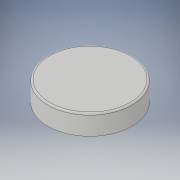
# Autodesk Inventor part: CCF
Saved by Autodesk Inventor 2018 (Build 220112000, 112)
## iProperties
Created: 2017-07-31
Part Number: CCF
Material: Generic
Document SubType Name: Modeling
Designer: Nour Kanso
Density: 1 g/cm^3
Appearance: Default
Author: Nour Kanso
Autodesk Inventor part; units mm, degrees
ref_plane "YZ Plane" through (0, 0, 0) normal (1, 0, 0) x (0, 1, 0)
ref_plane "XZ Plane" through (0, 0, 0) normal (0, 1, 0) x (-1, 0, 0)
ref_plane "XY Plane" through (0, 0, 0) normal (0, 0, 1) x (1, 0, 0)
sketch "Sketch5" plane through (0, 0, 0) normal (0, 1, 0) x (-1, 0, 0)
  circle A0 centre (0, 0) radius 32.131
  dimension "d28" = 64.262
  constraints: 1 centre point, 1 coincident
  measures "d28" diameter of A0
extrude "Extrusion3" add sketch "Sketch5" along normal blind 15.24
fillet "Fillet2" radius 1.27 1 edges at (32.131, 15.24, 0)
shell "Shell5" thickness 1.27 removed faces 1 at (-12.2357, 0, 10.0143)
thread "Thread6" size "2 1/2-4 UNC" class "2B" standard "ANSI Unified Screw Threads" full length
sketch "Sketch14" plane through (0, 13.97, 30.861) normal (-1, 0, 0) x (0, -1, 0)
  line L0 (-3.762, -0.339) -> (-3.1751, -0.339) construction
  line L1 (0.5868, -3.8052) -> (-0.0001, -4.8217) construction
  line L2 (-6.3501, -4.8217) -> (-6.937, -3.8052) construction
  line L3 (-2.5882, -0.339) -> (-3.1751, 0.6775) construction
  line L4 (-3.1751, 0.6775) -> (-3.762, -0.339) construction
  line L5 (-6.3501, -4.8217) -> (-5.7632, -3.8052) construction
  line L6 (-2.5882, -0.339) -> (-0.587, -3.8052)
  line L7 (-6.937, -3.8052) -> (-5.7632, -3.8052) construction
  arc A0 (-6.937, -3.8052) -> (-6.3501, -4.1441) centre (-6.3501, -3.4664) ccw construction
  line L8 (0.5868, -3.8052) -> (-0.587, -3.8052) construction
  line L9 (-6.3501, -4.8217) -> (-6.3501, -3.8052) construction
  line L10 (-0.0001, -4.8217) -> (-0.0001, -3.8052) construction
  line L11 (-3.1751, 0.6775) -> (-3.1751, -0.0002) construction
  line L12 (-6.3501, -4.1441) -> (-0.0001, -4.1441)
  arc A1 (-6.3501, -4.1441) -> (-5.7632, -3.8052) centre (-6.3501, -3.4664) ccw
  line L13 (-0.587, -3.8052) -> (-0.0001, -4.8217) construction
  line L14 (-5.7632, -3.8052) -> (-3.762, -0.339)
  line L15 (-0.0001, -0.0002) -> (-0.0001, 0.0177)
  line L16 (-0.0001, 0.0177) -> (-0.0001, -0.0002)
  line L17 (-0.0001, -0.0002) -> (0.0334, -0.0002)
  arc A2 (-0.587, -3.8052) -> (-0.0001, -4.1441) centre (-0.0001, -3.4664) ccw
  arc A3 (-0.0001, -4.1441) -> (0.5868, -3.8052) centre (-0.0001, -3.4664) ccw construction
  arc A4 (-3.1751, -0.0002) -> (-3.762, -0.339) centre (-3.1751, -0.6779) ccw
  arc A5 (-2.5882, -0.339) -> (-3.1751, -0.0002) centre (-3.1751, -0.6779) ccw
  line L18 (-3.1751, -0.0002) -> (-3.1751, -0.339) construction
  line L19 (-3.1751, -0.339) -> (-2.5882, -0.339) construction
  dimension "d117" = 60
  dimension "d118" = 1.0165
  dimension "d119" = 1.0165
  dimension "Sketch14_ThreadOffset" = 0
  dimension "Sketch14_MajorRadius" = 4.1439
  dimension "d122" = 6.35
  dimension "Sketch14_MinorRadius" = 0
  constraints: 40 end point, 12 point on circle, 10 parallel, 8 tangent, 6 centre point, 6 collinear, 2 midpoint, 2 point on line, 1 horizontal, 1 perpendicular, 3 other
  measures "d117" angle of L6 L14
  measures "d118" distance of L3.end L0.end
  measures "d119" distance of L1.end L10.end
  measures "Sketch14_ThreadOffset" distance between parallel lines of L15 L10
  measures "Sketch14_MajorRadius" distance from line of L12 L15.start
  measures "d122" distance from line of L1.end L9
  measures "Sketch14_MinorRadius" distance edge to line of A5 L17
sketch "Sketch15" plane through (0, 13.97, 0) normal (1, 0, 0) x (0, 0, 1)
  line L0 (30.861, 0) -> (30.861, 13.97)
  line L1 (30.861, 13.97) -> (26.7171, 13.97)
  line L2 (26.7171, 13.97) -> (26.7171, 0)
  line L3 (26.7171, 0) -> (30.861, 0)
  line L4 (0, -11.1729) -> (0, 18.1605) projected
  constraints: 8 end point
revolve "Revolution6" add sketch "Sketch15" angle 360 about axis through (0, 13.97, 0) along (0, -1, 0) separate body
coil "Coil6" sketch "Sketch14" operation cut axis through (0, 13.97, 0) along (0, -1, 0) pitch 6.35 turns 2 hand right bodies 2
equation "\"d117\" = d124"
equation "\"d118\" = 0.160083 * Sketch14_Pitch"
equation "\"d119\" = 0.160083 * Sketch14_Pitch"
equation "\"d122\" = Sketch14_Pitch"
equation "\"d14\" = 60deg"
equation "\"Sketch2_Pitch\" = 6.35"
equation "\"d42\" = 60deg"
equation "\"Sketch6_Pitch\" = 6.35"
equation "\"d62\" = 60deg"
equation "\"Sketch8_Pitch\" = 6.35"
equation "\"d82\" = 60deg"
equation "\"Sketch10_Pitch\" = 6.35"
equation "\"d103\" = 60deg"
equation "\"Sketch12_Pitch\" = 4.23333"
equation "\"d124\" = 60deg"
equation "\"Sketch14_Pitch\" = 6.35"
body "Solid3"
body "Solid8"
